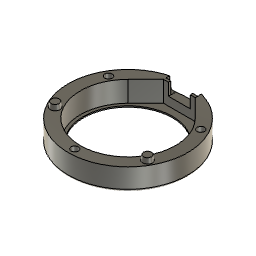
frontpiece (Autodesk Fusion 360 design; units mm, degrees)
Autodesk Fusion 360 part; units mm, degrees
sketch "Sketch1" plane through (0, 0, 0) normal (0, 0, 1) x (1, 0, 0)
  circle A0 centre (18.006673, 0) radius 19.5
  circle A1 centre (18.006673, 0) radius 18.25
  line L0 (18.006673, 0) -> (18.006673, 21.961283) construction
  line L1 (0, 0) -> (17.983384, 0) construction
  circle A2 centre (18.006673, 0) radius 24.5
  line L2 (11.751541, 20.51766) -> (14.461598, 20.51766) construction
  line L3 (11.506673, 21.07716) -> (11.506673, 23.622024)
  line L4 (-6.493327, 0) -> (46.000001, 0) construction
  line L5 (45.000001, -5) -> (-3, -5) construction
  line L6 (18.006673, 17.406836) -> (18.006673, -16.288718) construction
  line L7 (23.006673, 5.711283) -> (23.006673, -8.288717) construction
  line L8 (18.006673, 0) -> (35.339937, 17.333263) construction
  line L9 (18.006673, 0) -> (42.723763, 0) construction
  line L10 (17.983384, 0) -> (-3.229819, 21.213203) construction
  line L11 (17.983384, 0) -> (37.467715, 0) construction
  line L12 (31.795256, 13.788582) -> (24.506673, 21.077164)
  line L13 (11.506673, 21.07716) -> (4.206451, 13.776933)
  line L14 (24.506673, 23.622024) -> (24.506673, 21.077164)
  line L15 (24.506673, 21.077164) -> (11.506673, 21.07716)
  dimension "d1" = 39
  dimension "d7" = 36.5
  dimension "d15" = 90
  dimension "d22" = 49
  dimension "d95" = 5
  dimension "d96" = 5
  dimension "d97" = 5
  dimension "d98" = 5
  dimension "d100" = 5
  dimension "d101" = 5
  dimension "d102" = 5
  dimension "d103" = 5
  dimension "d104" = 45
  dimension "d105" = 5
  dimension "d106" = 5
  dimension "d107" = 135
  dimension "d108" = 90
  dimension "d109" = 30
  dimension "d114" = 13
  dimension "d115" = 6.5
  constraint vertical L0
  constraint coincident L1.start origin
  constraint concentric A1 A2
  constraint horizontal L2
  constraint perpendicular L2 L3
  constraint horizontal L4
  constraint parallel L4 L5
  constraint vertical L6
  constraint perpendicular L4 L7
  constraint horizontal L9
  constraint horizontal L11
  constraint tangent A0 L12
  constraint vertical L14
  measures "d1" diameter of A0
  measures "d7" diameter of A1
  measures "d15" angle of L0 L1
  measures "d22" diameter of A2
  measures "d95" distance of L4 L5
  measures "d101" distance of L6 L7
  measures "d104" angle of L8 L9
  measures "d105" distance of L5 L9
  measures "d106" distance of L1 L5
  measures "d107" angle of L10 L11
  measures "d108" angle of L8 L10
  measures "d114" distance of L3 L14
  measures "d115" distance of L0 L3
other "Base Mesh Feature1"
extrude "Extrude1" add sketch "Sketch1" along normal blind 8 contours A0 A2 L3 L12 L13 L14 picked at (6.868893, 18.51647) makes body 1
extrude "Extrude19" add sketch "Sketch1" along normal blind 3 contours A2 L3 L14 L15 picked at (18.006673, 22.218108) bodies 1
extrude "Extrude2" add sketch "Sketch1" against normal blind 1 contours A0 A2 L3 L12 L13 L14 | A2 L3 L14 L15 picked at (6.868893, 18.51647) picked at (18.006673, 22.218108) bodies 1
extrude "Extrude3" add sketch "Sketch1" along normal blind 0.5 from surface at -1 contours A0 L12 L13 L15 picked at (17.552065, 20.117765) bodies 1
other "Modify1"
fillet "Fillet1" radius 1 1 edges at (-4.835347, 8.859578, -1) on bodies 1
sketch "Sketch11" plane through (-0.000008, 21.077156, 0) normal (0, -1, 0) x (1, 0, 0)
  line L0 (11.506681, -0.5) -> (24.506681, -0.5)
  line L1 (24.506681, -0.5) -> (24.506681, 3)
  line L2 (24.506681, 3) -> (11.506681, 3)
  line L3 (11.506681, 3) -> (11.506681, -0.5)
  line L4 (13.506681, 4) -> (13.506681, 6)
  line L5 (22.506681, 6) -> (22.506681, 4)
  line L6 (24.506681, 4) -> (24.506681, 6)
  line L7 (24.506681, 6) -> (22.506681, 6)
  line L8 (22.506681, 6) -> (22.506681, 4)
  line L9 (11.506681, 4) -> (11.506681, 6)
  line L10 (11.506681, 6) -> (13.506681, 6)
  line L11 (13.506681, 6) -> (13.506681, 4)
  line L12 (24.506681, 4) -> (24.506681, 3)
  line L13 (24.506681, 3) -> (22.506681, 3)
  line L14 (22.506681, 3) -> (22.506681, 4)
  line L15 (11.506681, 4) -> (11.506681, 3)
  line L16 (11.506681, 3) -> (13.506681, 3)
  line L17 (13.506681, 3) -> (13.506681, 4)
  line L18 (22.506681, 6) -> (24.506681, 6)
  line L19 (24.506681, 6) -> (24.506681, 4)
  line L20 (24.506681, 4) -> (22.506681, 4)
  line L21 (22.506681, 4) -> (22.506681, 6)
  line L22 (13.506681, 6) -> (11.506681, 6)
  line L23 (11.506681, 6) -> (11.506681, 4)
  line L24 (11.506681, 4) -> (13.506681, 4)
  line L25 (13.506681, 4) -> (13.506681, 6)
  line L26 (22.506681, 6) -> (24.5, 6)
  line L27 (24.5, 6) -> (24.5, 8)
  line L28 (24.5, 8) -> (22.506681, 8)
  line L29 (22.506681, 8) -> (22.506681, 6)
  line L30 (13.506681, 6) -> (11.506681, 6)
  line L31 (11.506681, 6) -> (11.506681, 8)
  line L32 (11.506681, 8) -> (13.506681, 8)
  line L33 (13.506681, 8) -> (13.506681, 6)
  dimension "d150" = 9
  dimension "d153" = 2
  dimension "d154" = 2
  dimension "d155" = 2
  dimension "d156" = 2
  dimension "d163" = 2
  dimension "d164" = 2
  dimension "d165" = 2
  constraint vertical L4
  constraint vertical L5
  constraint vertical L6
  constraint horizontal L7
  constraint vertical L8
  constraint vertical L9
  constraint horizontal L10
  constraint vertical L11
  constraint vertical L12
  constraint horizontal L13
  constraint vertical L14
  constraint vertical L15
  constraint horizontal L16
  constraint vertical L17
  constraint horizontal L18
  constraint vertical L19
  constraint horizontal L20
  constraint vertical L21
  constraint horizontal L22
  constraint vertical L23
  constraint horizontal L24
  constraint vertical L25
  constraint horizontal L26
  constraint vertical L27
  constraint horizontal L28
  constraint vertical L29
  constraint horizontal L30
  constraint vertical L31
  constraint horizontal L32
  constraint vertical L33
  measures "d153" distance of L3 L4
  measures "d154" distance of L1 L5
extrude "Extrude22" add sketch "Sketch11" against normal blind 1 contours L2 L15 L16 L17 L24 | L2 L12 L13 L14 L20 | L4 L9 L10 L11 L22 L23 L24 L25 L30 | L5 L6 L7 L8 L18 L19 L20 L21 L26 | L10 L22 L30 L31 L32 L33 | L7 L18 L26 L27 L28 L29 picked at (12.173347, 3.333333) picked at (23.840014, 3.333333) picked at (12.173347, 5.333333) picked at (23.837787, 4.666667) picked at (12.840014, 6.666667) picked at (23.171121, 7.333333) bodies 1
extrude "Extrude23" add sketch "Sketch11" against normal blind 2.5 from surface at 41 contours L4 L9 L10 L11 L22 L23 L24 L25 L30 | L5 L6 L7 L8 L18 L19 L20 L21 L26 picked at (12.173347, 5.333333) picked at (23.837787, 4.666667) bodies 1
sketch "Sketch2" plane through (0, 0, 8) normal (0, 0, 1) x (-1, 0, 0)
  arc A0 (-4.206451, -13.776933) -> (-31.795256, -13.788582) centre (-18.006673, 0) ccw
  arc A1 (-11.506673, -23.622024) -> (-24.506673, -23.622024) centre (-18.006673, 0) ccw
  circle A2 centre (-18.006673, 0) radius 24.5
  circle A3 centre (-17.996047, -0.019742) radius 18.256337
  circle A4 centre (-17.996047, -0.019742) radius 21.875 construction
  line L0 (-25.506673, 22) -> (-10.506673, 22) construction
  line L1 (-10.506673, 22) -> (-10.506673, 18.513429) construction
  line L2 (-10.506673, 18.513429) -> (-25.506673, 18.513429) construction
  line L3 (-25.506673, 18.513429) -> (-25.506673, 22) construction
  line L4 (-18.006673, 0) -> (-18.006673, 31) construction
  line L5 (-25.506673, 20.584016) -> (-25.506673, 19.524461)
  line L6 (-10.506673, 19.481161) -> (-10.506673, 20.549103)
  circle A5 centre (-18.006673, 21.855255) radius 1.5
  line L7 (-17.996047, -0.019742) -> (3.205055, -12.260204) construction
  line L8 (-17.996047, -0.019742) -> (6.516616, -0.019742) construction
  line L9 (-17.996047, -0.019742) -> (-39.195623, -12.259324) construction
  circle A6 centre (-36.940353, -10.957242) radius 1.5
  circle A7 centre (0.948259, -10.957242) radius 1.5
  line L10 (-17.996047, -0.019742) -> (3.222146, 12.230587) construction
  line L11 (-17.996047, -0.019742) -> (6.516616, -0.019742) construction
  line L12 (-17.996047, -0.019742) -> (-39.230185, 12.239793) construction
  circle A8 centre (-36.940353, 10.917758) radius 2
  circle A9 centre (0.948259, 10.917758) radius 2
  line L13 (-17.996047, -0.019742) -> (-10.496047, -0.019742)
  circle A10 centre (-10.496047, -0.019742) radius 3.5
  line L14 (-24.506673, -23.622024) -> (-24.506673, -21.077164)
  line L15 (-24.506673, -21.077164) -> (-31.795256, -13.788582)
  line L16 (-4.206451, -13.776933) -> (-11.506673, -21.07716)
  line L17 (-24.506673, -21.077164) -> (-11.506673, -21.07716)
  line L18 (-11.506673, -21.07716) -> (-13.506673, -21.077161)
  line L19 (-13.506673, -21.077161) -> (-13.506673, -22.077161)
  line L20 (-13.506673, -22.077161) -> (-11.506673, -22.07716)
  point P0 (-17.983384, 0)
  dimension "d26" = 49
  dimension "d28" = 36.512673
  dimension "d29" = 43.75
  dimension "d60" = 15
  dimension "d61" = 7.5
  dimension "d62" = 3
  dimension "d71" = 30
  dimension "d72" = 60
  dimension "d73" = 3
  dimension "d74" = 3
  dimension "d75" = 30
  dimension "d76" = 60
  dimension "d77" = 4
  dimension "d78" = 4
  dimension "d92" = 7.5
  dimension "d93" = 7
  constraint concentric A0 A2
  constraint concentric A3 A4
  constraint horizontal L0
  constraint vertical L1
  constraint horizontal L2
  constraint vertical L3
  constraint perpendicular L2 L4
  constraint horizontal L8
  constraint horizontal L11
  constraint parallel L8 L13
  measures "d26" diameter of A2
  measures "d28" diameter of A3
  measures "d29" diameter of A4
  measures "d61" distance of L3 L4
  measures "d62" diameter of A5
  measures "d71" angle of L7 L8
  measures "d72" angle of L7 L9
  measures "d73" diameter of A6
  measures "d74" diameter of A7
  measures "d75" angle of L10 L11
  measures "d76" angle of L10 L12
  measures "d77" diameter of A8
  measures "d78" diameter of A9
  measures "d93" diameter of A10
extrude "Extrude10" cut sketch "Sketch2" against normal blind 4 contours A5 | A6 | A7 picked at (-18.256673, 22.851588) picked at (-36.59604, -10.764534) picked at (0.827333, -10.533902) bodies 1
extrude "Extrude11" add sketch "Sketch2" along normal blind 2 draft -10 contours A8 | A9 picked at (-37.187227, 11.58256) picked at (0.799912, 11.56771) bodies 1
sketch "Sketch3" plane through (0, 0, 8) normal (0, 0, 1) x (-1, 0, 0)
  circle A0 centre (-17.983384, 0) radius 24.5
  circle A1 centre (-17.983384, 0) radius 18.25
  line L0 (-17.983384, 0) -> (-17.983384, 31) construction
  line L1 (-17.983384, 24.5) -> (-17.983384, 18.25) construction
  circle A2 centre (-17.983384, 21.375) radius 2
  arc A3 (-4.206451, -13.776933) -> (-31.795256, -13.788582) centre (-18.006673, 0) ccw
  line L2 (-11.506673, -22.07716) -> (-11.506673, -23.622024)
  circle A4 centre (0.948259, 10.917758) radius 2
  circle A5 centre (-36.940353, 10.917758) radius 2
  circle A6 centre (-18.006673, 21.855255) radius 1.5
  circle A7 centre (0.948259, -10.957242) radius 1.5
  circle A8 centre (-36.940353, -10.957242) radius 1.5
  circle A9 centre (0.948259, -10.957242) radius 1.05
  circle A10 centre (-36.940353, -10.957242) radius 1.05
  circle A11 centre (-18.006673, 21.855255) radius 1.05
  line L3 (-24.506673, -23.622024) -> (-24.506673, -21.077164)
  line L4 (-24.506673, -21.077164) -> (-31.795256, -13.788582)
  line L5 (-4.206451, -13.776933) -> (-11.506673, -21.07716)
  line L6 (-24.506673, -21.077164) -> (-11.506673, -22.07716)
  line L7 (-24.506673, -21.077164) -> (-24.506673, -23.622024)
  line L8 (-11.506673, -22.07716) -> (-11.506673, -23.622024)
  arc A12 (-24.506673, -23.622024) -> (-11.506673, -23.622024) centre (-18.006673, 0) ccw
  line L9 (-11.506673, -21.07716) -> (-13.506673, -21.077161)
  line L10 (-13.506673, -21.077161) -> (-13.506673, -22.077161)
  line L11 (-13.506673, -22.077161) -> (-11.506673, -22.07716)
  point P0 (-17.983384, 0)
  point P1 (-17.983384, 0)
  dimension "d34" = 49
  dimension "d35" = 36.5
  dimension "d67" = 4
  dimension "d87" = 2.1
  dimension "d88" = 2.1
  dimension "d89" = 2.1
  constraint vertical L0
  constraint concentric A7 A9
  constraint concentric A8 A10
  constraint concentric A6 A11
  measures "d34" diameter of A0
  measures "d35" diameter of A1
  measures "d67" diameter of A2
  measures "d87" diameter of A9
  measures "d88" diameter of A10
  measures "d89" diameter of A11
extrude "Extrude6" add sketch "Sketch3" along normal blind 6 separate body contours A0 A2 A3 L2 L3 L4 L5 L6 L7 L8 A12 L9 L10 | A0 L2 L3 L6 L7 L8 A12 L10 L11 | A0 L3 L7 A12 | A2 A3 L4 L5 L6 L9 L10 | L6 L10 L11 | A2 A3 | A2 A3 | A4 | A5 | A6 | A7 | A8 | A9 | A10 | A11 picked at (-29.139158, -18.516329) picked at (-18.669458, -22.500159) picked at (-23.792953, -23.780847) picked at (-19.120185, -20.399816) picked at (-12.840006, -22.025878) picked at (-17.94034, 19.458967) picked at (-18.399171, 19.793739) picked at (0.799912, 11.56771) picked at (-37.187227, 11.58256) picked at (-16.666167, 21.728569) picked at (2.292674, -11.031764) picked at (-36.518552, -12.235949) picked at (1.237442, -10.76008) picked at (-37.100837, -10.196214) picked at (-17.72395, 21.744294) makes body 2
extrude "Extrude20" cut sketch "Sketch3" along normal blind 2 contours A0 L2 L3 L6 L7 L8 A12 L10 L11 | A0 L3 L7 A12 | L6 L10 L11 picked at (-18.669458, -22.500159) picked at (-23.792953, -23.780847) picked at (-12.840006, -22.025878) bodies 2
move_body "Move1" bodies 1 to x (1, 0, 0) y (0, 1, 0) z (0, 0, 1) at (0, 0, -5)
extrude "Extrude14" add sketch "Sketch2" along normal blind 1 contours A0 L15 L16 L17 L18 | A3 picked at (-19.124564, -20.126452) picked at (-28.765635, 0.887246) bodies 2
extrude "Extrude12" cut sketch "Sketch3" along normal blind 8 contours A9 | A10 | A11 picked at (1.237442, -10.76008) picked at (-37.100837, -10.196214) picked at (-17.72395, 21.744294) bodies 2
extrude "Extrude13" cut sketch "Sketch3" along normal blind 2 draft -10 contours A4 | A5 picked at (0.799912, 11.56771) picked at (-37.187227, 11.58256) bodies 2
sketch "Sketch4" plane through (0, 0, 26) normal (0, 0, 1) x (-1, 0, 0)
  circle A0 centre (-36.940353, -10.957242) radius 1.05
  circle A1 centre (0.948259, -10.957242) radius 1.05
  circle A2 centre (-18.006673, 21.855255) radius 1.05
  circle A3 centre (-17.983384, 0) radius 18.25
  circle A4 centre (-17.983384, 0) radius 24.5
  circle A5 centre (-17.983384, 0) radius 24.5
  circle A6 centre (-17.983384, 0) radius 18.25
  circle A7 centre (-18.006673, 21.855255) radius 1.05
  circle A8 centre (0.948259, -10.957242) radius 1.05
  circle A9 centre (-36.940353, -10.957242) radius 1.05
  constraint concentric A3 A5
  constraint concentric A3 A6
  constraint concentric A2 A7
  constraint concentric A1 A8
  constraint concentric A0 A9
extrude "Extrude15" add sketch "Sketch4" along normal blind 1 separate body contours A3 A6 | A4 A5 picked at (-19.939492, -8.570271) picked at (2.071945, -7.52687) makes body 3
extrude "Extrude16" add sketch "Sketch4" against normal blind 3 contours A4 A5 picked at (2.071945, -7.52687) bodies 3
chamfer "Chamfer2" distance 1.3 angle 45 3 edges at (18.985617, -22.234951, 27) (0.030685, 10.577546, 27) (37.919296, 10.577546, 27) on bodies 3
sketch "Sketch6" plane through (0, 0, 23) normal (0, 0, -1) x (1, 0, 0)
  circle A0 centre (-0.948259, -10.957242) radius 1.05
  circle A1 centre (17.983384, 0) radius 18.25
  circle A2 centre (18.006673, 21.855255) radius 1.05
  circle A3 centre (36.940353, -10.957242) radius 1.05
  circle A4 centre (17.983384, 0) radius 24.5
sketch "Sketch7" plane through (0, 0, 0) normal (0, 1, 0) x (1, 0, 0)
  line L0 (-6.02823, -25) -> (-6.52823, -25)
  line L1 (-6.52823, -25) -> (-6.52823, -23)
  line L2 (-6.52823, -23) -> (-6.02823, -23)
  line L3 (-6.02823, -23) -> (-6.02823, -25)
  line L4 (-6.516616, -27) -> (42.483384, -27)
  dimension "d136" = 0.5
  dimension "d137" = 2
  dimension "d139" = 2
  constraint horizontal L0
  constraint vertical L1
  constraint horizontal L2
  constraint vertical L3
  measures "d139" distance of L0 L4
revolve "Revolve2" cut sketch "Sketch7" angle 360 about axis through (17.983384, 0, 26) along (0, 0, -1) contours L0 L1 L2 L3 picked at (-6.194897, -24.333333) bodies 3
delete_face "DeleteFace1" 1 faces at (14.360222, 24.227121, 9.333333) on bodies 2
fillet "Fillet3" radius 2 2 edges at (24.506673, 22.849594, -2) (11.506673, 22.849592, -2) on bodies 1 2
fillet "Fillet3" radius 2 2 edges at (24.506673, 22.346384, 10) (11.506673, 22.85279, 10) on bodies 1 2
other "Base Mesh Feature3"
other "Modify2"
move_body "Move2" bodies 1 to x (1, 0, 0) y (0, 1, 0) z (0, 0, 1) at (0, 0, -6)
other "Modify3"
other "Modify4"
move_body "Move3" bodies 2 to x (1, 0, 0) y (0, 1, 0) z (0, 0, 1) at (0, 0, -11)
other "Modify5"
other "Modify6"
other "Modify7"
other "Modify8"
hidden bodies 2 3
